Antennastandend (Autodesk Fusion 360 design; units mm, degrees)
Autodesk Fusion 360 part; units mm, degrees
sketch "Sketch1" plane through (0, 0, 0) normal (0, 1, 0) x (1, 0, 0)
  line L0 (0, 0) -> (0, -70)
  line L1 (12.55, 0) -> (12.55, -20)
  line L2 (13.95, 0) -> (13.95, -20)
  line L3 (12.55, -20) -> (2.55, -30)
  line L4 (12.55, -20) -> (30.2984, -20) construction
  line L5 (13.95, -20) -> (0.4722, -33.4778)
  line L6 (0, -30) -> (2.55, -30)
  line L7 (12.55, 0) -> (13.95, 0)
  line L8 (0, -33.95) -> (0, -30)
  circle A0 centre (21.45, -10) radius 2.5
  line L9 (28.95, -10) -> (28.95, -15)
  line L10 (28.95, -10) -> (28.95, -5)
  line L11 (13.95, -20) -> (28.95, -15)
  line L12 (28.95, -5) -> (13.95, 0)
  line L13 (13.6343, -20) -> (13.6343, 0)
  line L14 (13.95, -20) -> (13.6343, -20)
  line L15 (13.95, 0) -> (13.6343, 0)
  line L16 (0, -33.4778) -> (0.4722, -33.4778)
  dimension "d1" = 20
  dimension "d2" = 12.55
  dimension "d3" = -1.4
  dimension "d4" = 135
  dimension "d6" = 5
  dimension "d7" = 7.5
  dimension "d8" = 7.5
  dimension "d9" = 5
  constraint coincident L0.start origin
  constraint vertical L0
  constraint parallel L0 L1
  constraint horizontal L4
  constraint coincident L0 L8.start
  constraint parallel L3 L5
  constraint coincident L0 L6.start
  constraint perpendicular L0 L6
  constraint perpendicular L1 L7
  constraint coincident L4 L13.start
  constraint coincident L7 L13.end
  constraint perpendicular L7 L13
  constraint perpendicular L13 L14
  constraint coincident L0 L16.start
  constraint perpendicular L0 L16
  measures "d1" distance of L1.start L1.end
  measures "d2" distance of L0 L1
  measures "d4" angle of L3 L4
  measures "d6" diameter of A0
  measures "d7" distance of L2 A0.centre
  measures "d8" distance of A0.centre L9.start
  measures "d9" distance of L9.start L9.end
revolve "Revolve1" add sketch "Sketch1" angle 360 about axis through (0, 0, 0) along (0, 0, 1) contours L0 L1 L3 L5 L6 L7 L8 L13 L14 L16 | L2 L7 L13 L14 L15
extrude "Extrude2" add sketch "Sketch1" along normal mid plane 2.4 contours L2 L7 L13 L14 L15 | L2 L9 L10 L11 L12
chamfer "Chamfer1" distance 2 angle 45 2 edges at (13.8983, -1.2, 10) (13.8983, 1.2, 10)
fillet "Fillet2" radius 7 2 edges at (28.95, 0, 15) (28.95, 0, 5)
